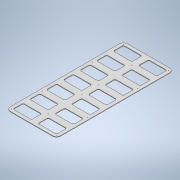
# Autodesk Inventor part: front_Box
Saved by Autodesk Inventor 2020 (Build 240168000, 168)
## iProperties
Created: 2020-07-08
Part Number: front_Box
Material: Generic
Document SubType Name: Modeling
Designer: gerac
Density: 1 g/cm^3
Appearance: Default
Author: gerac
Autodesk Inventor part; units mm, degrees
ref_plane "YZ Plane" through (0, 0, 0) normal (1, 0, 0) x (0, 1, 0)
ref_plane "XZ Plane" through (0, 0, 0) normal (0, 1, 0) x (-1, 0, 0)
ref_plane "XY Plane" through (0, 0, 0) normal (0, 0, 1) x (1, 0, 0)
sketch "Sketch1" plane through (0, 0, 0) normal (0, 1, 0) x (-1, 0, 0)
  line L0 (144, 336) -> (-144, 336)
  line L1 (-144, 336) -> (-144, -336)
  line L2 (-144, -336) -> (144, -336)
  line L3 (144, -336) -> (144, 336)
  line L4 (144, 336) -> (-144, -336) construction
  line L5 (-144, 336) -> (144, -336) construction
  line L6 (-24, 317) -> (-19, 312)
  line L7 (-19, 264) -> (-24, 259)
  line L8 (-125, 264) -> (-120, 259)
  line L9 (-120, 317) -> (-125, 312)
  line L10 (-19, 312) -> (-19, 264)
  line L11 (-24, 259) -> (-120, 259)
  line L12 (-24, 317) -> (-120, 317)
  line L13 (-125, 312) -> (-125, 264)
  line L14 (-24, 221) -> (-120, 221)
  line L15 (-24, 221) -> (-19, 216)
  line L16 (-19, 216) -> (-19, 168)
  line L17 (-24, 163) -> (-120, 163)
  line L18 (-19, 168) -> (-24, 163)
  line L19 (-125, 168) -> (-120, 163)
  line L20 (-125, 216) -> (-125, 168)
  line L21 (-120, 221) -> (-125, 216)
  line L22 (-24, 125) -> (-120, 125)
  line L23 (-24, 125) -> (-19, 120)
  line L24 (-19, 120) -> (-19, 72)
  line L25 (-24, 67) -> (-120, 67)
  line L26 (-19, 72) -> (-24, 67)
  line L27 (-125, 72) -> (-120, 67)
  line L28 (-125, 120) -> (-125, 72)
  line L29 (-120, 125) -> (-125, 120)
  line L30 (-24, 29) -> (-120, 29)
  line L31 (-24, 29) -> (-19, 24)
  line L32 (-19, 24) -> (-19, -24)
  line L33 (-24, -29) -> (-120, -29)
  line L34 (-19, -24) -> (-24, -29)
  line L35 (-125, -24) -> (-120, -29)
  line L36 (-125, 24) -> (-125, -24)
  line L37 (-120, 29) -> (-125, 24)
  line L38 (-24, -67) -> (-120, -67)
  line L39 (-24, -67) -> (-19, -72)
  line L40 (-19, -72) -> (-19, -120)
  line L41 (-24, -125) -> (-120, -125)
  line L42 (-19, -120) -> (-24, -125)
  line L43 (-125, -120) -> (-120, -125)
  line L44 (-125, -72) -> (-125, -120)
  line L45 (-120, -67) -> (-125, -72)
  line L46 (-24, -163) -> (-120, -163)
  line L47 (-24, -163) -> (-19, -168)
  line L48 (-19, -168) -> (-19, -216)
  line L49 (-24, -221) -> (-120, -221)
  line L50 (-19, -216) -> (-24, -221)
  line L51 (-125, -216) -> (-120, -221)
  line L52 (-125, -168) -> (-125, -216)
  line L53 (-120, -163) -> (-125, -168)
  line L54 (-24, -259) -> (-120, -259)
  line L55 (-24, -259) -> (-19, -264)
  line L56 (-19, -264) -> (-19, -312)
  line L57 (-24, -317) -> (-120, -317)
  line L58 (-19, -312) -> (-24, -317)
  line L59 (-125, -312) -> (-120, -317)
  line L60 (-125, -264) -> (-125, -312)
  line L61 (-120, -259) -> (-125, -264)
  line L62 (120, 317) -> (24, 317)
  line L63 (120, 317) -> (125, 312)
  line L64 (125, 312) -> (125, 264)
  line L65 (120, 259) -> (24, 259)
  line L66 (125, 264) -> (120, 259)
  line L67 (19, 264) -> (24, 259)
  line L68 (19, 312) -> (19, 264)
  line L69 (24, 317) -> (19, 312)
  line L70 (120, 221) -> (24, 221)
  line L71 (120, 221) -> (125, 216)
  line L72 (125, 216) -> (125, 168)
  line L73 (120, 163) -> (24, 163)
  line L74 (125, 168) -> (120, 163)
  line L75 (19, 168) -> (24, 163)
  line L76 (19, 216) -> (19, 168)
  line L77 (24, 221) -> (19, 216)
  line L78 (120, 125) -> (24, 125)
  line L79 (120, 125) -> (125, 120)
  line L80 (125, 120) -> (125, 72)
  line L81 (120, 67) -> (24, 67)
  line L82 (125, 72) -> (120, 67)
  line L83 (19, 72) -> (24, 67)
  line L84 (19, 120) -> (19, 72)
  line L85 (24, 125) -> (19, 120)
  line L86 (120, 29) -> (24, 29)
  line L87 (120, 29) -> (125, 24)
  line L88 (125, 24) -> (125, -24)
  line L89 (120, -29) -> (24, -29)
  line L90 (125, -24) -> (120, -29)
  line L91 (19, -24) -> (24, -29)
  line L92 (19, 24) -> (19, -24)
  line L93 (24, 29) -> (19, 24)
  line L94 (120, -67) -> (24, -67)
  line L95 (120, -67) -> (125, -72)
  line L96 (125, -72) -> (125, -120)
  line L97 (120, -125) -> (24, -125)
  line L98 (125, -120) -> (120, -125)
  line L99 (19, -120) -> (24, -125)
  line L100 (19, -72) -> (19, -120)
  line L101 (24, -67) -> (19, -72)
  line L102 (120, -163) -> (24, -163)
  line L103 (120, -163) -> (125, -168)
  line L104 (125, -168) -> (125, -216)
  line L105 (120, -221) -> (24, -221)
  line L106 (125, -216) -> (120, -221)
  line L107 (19, -216) -> (24, -221)
  line L108 (19, -168) -> (19, -216)
  line L109 (24, -163) -> (19, -168)
  line L110 (120, -259) -> (24, -259)
  line L111 (120, -259) -> (125, -264)
  line L112 (125, -264) -> (125, -312)
  line L113 (120, -317) -> (24, -317)
  line L114 (125, -312) -> (120, -317)
  line L115 (19, -312) -> (24, -317)
  line L116 (19, -264) -> (19, -312)
  line L117 (24, -259) -> (19, -264)
  point P0 (0, 0)
  dimension "d0" = 288
  dimension "d1" = 672
  dimension "d19" = 19
  dimension "d30" = 48
  dimension "d31" = 58
  dimension "d32" = 96
  dimension "d33" = 106
  dimension "d34" = 19
  dimension "d38" = 5
  dimension "d39" = 5
  dimension "d40" = 5
  dimension "d41" = 5
  dimension "d42" = 5
  dimension "d43" = 5
  dimension "d44" = 5
  dimension "d47" = 96
  dimension "d50" = 144
  constraints: 236 end point, 14 point on line, 3 vertical, 2 horizontal, 2 midpoint, 2 parallel, 2 perpendicular, 221 other
  measures "d0" distance of L2.end L1.end
  measures "d1" distance of L1.end L0.end
  measures "d19" distance between parallel lines of L0 L12
  measures "d30" distance of L6.end L10.end
  measures "d31" distance between parallel lines of L11 L12
  measures "d32" distance of L7.end L8.end
  measures "d33" distance between parallel lines of L13 L10
  measures "d34" distance between parallel lines of L1 L13
  measures "d38" horizontal distance of L8.start L8.end
  measures "d39" horizontal distance of L8.start L8.end
  measures "d40" horizontal distance of L9.start L9.end
  measures "d41" horizontal distance of L9.start L9.end
  measures "d42" horizontal distance of L6.start L6.end
  measures "d43" horizontal distance of L6.start L6.end
  measures "d44" horizontal distance of L7.start L7.end
  measures "d47" distance of L6.start L14.start
  measures "d50" distance of L6.start L62.start
extrude "Extrusion2" add sketch "Sketch1" along normal blind 3
fillet "Fillet1" radius 24 4 edges at (-144, 1.5, 336) (-144, 1.5, -336) (144, 1.5, 336) (144, 1.5, -336)
sketch "Sketch3" plane through (0, 3, 0) normal (0, 1, 0) x (1, 0, 0)
  circle A0 centre (0, -240) radius 1.25
  line L0 (-120, -336) -> (120, -336) projected
  line L1 (144, -312) -> (144, 312) projected
  circle A1 centre (0, -48) radius 1.25
  circle A2 centre (0, 48) radius 1.25
  circle A3 centre (0, 240) radius 1.25
  point P0 (0, 0)
  dimension "d85" = 2.5
  dimension "d86" = 96
  dimension "d87" = 144
  dimension "d88" = 2.5
  dimension "d89" = 2.5
  dimension "d90" = 2.5
  dimension "d91" = 192
  dimension "d92" = 144
  dimension "d93" = 96
  dimension "d94" = 144
  dimension "d95" = 192
  dimension "d96" = 144
  constraints: 4 centre point
  measures "d85" diameter of A0
  measures "d86" distance from line of L0 A0.centre
  measures "d87" distance from line of L1 A0.centre
  measures "d88" diameter of A1
  measures "d89" diameter of A2
  measures "d90" diameter of A3
  measures "d91" distance of A0.centre A1.centre
  measures "d92" distance from line of L1 A1.centre
  measures "d93" distance of A1.centre A2.centre
  measures "d94" distance from line of L1 A2.centre
  measures "d95" distance of A2.centre A3.centre
  measures "d96" distance from line of L1 A3.centre
extrude "Extrusion4" cut sketch "Sketch3" against normal blind 10
sketch "Sketch4" plane through (0, 3, 0) normal (0, 1, 0) x (1, 0, 0)
  circle A0 centre (-130, -144) radius 1.25
  circle A1 centre (130, -144) radius 1.25
  circle A2 centre (-130, -322) radius 1.25
  circle A3 centre (130, -322) radius 1.25
  circle A4 centre (-130, 144) radius 1.25
  circle A5 centre (-130, 322) radius 1.25
  circle A6 centre (130, 144) radius 1.25
  circle A7 centre (130, 322) radius 1.25
  line L0 (144, -312) -> (144, 312) projected
  line L1 (-120, -336) -> (120, -336) projected
  line L2 (125, -312) -> (120, -317) projected
  line L3 (24, -163) -> (120, -163) projected
  line L4 (-144, 312) -> (-144, -312) projected
  line L5 (-120, -163) -> (-24, -163) projected
  line L6 (-120, 125) -> (-24, 125) projected
  line L7 (24, 125) -> (120, 125) projected
  line L8 (120, 317) -> (125, 312) projected
  line L9 (-125, 312) -> (-120, 317) projected
  line L10 (120, 336) -> (-120, 336) projected
  line L11 (-120, -317) -> (-125, -312) projected
  point P0 (0, 0)
  dimension "d99" = 2.5
  dimension "d100" = 2.5
  dimension "d101" = 2.5
  dimension "d102" = 2.5
  dimension "d104" = 2.5
  dimension "d105" = 2.5
  dimension "d106" = 2.5
  dimension "d107" = 2.5
  dimension "d112" = 14
  dimension "d113" = 19
  dimension "d114" = 14
  dimension "d115" = 19
  dimension "d116" = 19
  dimension "d117" = 14
  dimension "d118" = 14
  dimension "d119" = 19
  dimension "d129" = 14
  dimension "d130" = 14
  dimension "d131" = 14
  dimension "d132" = 14
  dimension "d133" = 14
  dimension "d134" = 14
  dimension "d135" = 14
  dimension "d136" = 14
  constraints: 8 centre point
  measures "d99" diameter of A0
  measures "d100" diameter of A1
  measures "d101" diameter of A2
  measures "d102" diameter of A3
  measures "d104" diameter of A4
  measures "d105" diameter of A5
  measures "d106" diameter of A6
  measures "d107" diameter of A7
  measures "d112" distance from line of L0 A1.centre
  measures "d113" distance from line of L3 A1.centre
  measures "d114" distance from line of L4 A0.centre
  measures "d115" distance from line of L5 A0.centre
  measures "d116" distance from line of L6 A4.centre
  measures "d117" distance from line of L4 A4.centre
  measures "d118" distance from line of L0 A6.centre
  measures "d119" distance from line of L7 A6.centre
  measures "d129" distance from line of A3.centre L1
  measures "d130" distance from line of L0 A3.centre
  measures "d131" distance from line of A7.centre L10
  measures "d132" distance from line of L0 A7.centre
  measures "d133" distance from line of L4 A5.centre
  measures "d134" distance from line of L10 A5.centre
  measures "d135" distance from line of L4 A2.centre
  measures "d136" distance from line of L1 A2.centre
extrude "Extrusion5" cut sketch "Sketch4" against normal blind 3
body "Solid2"
